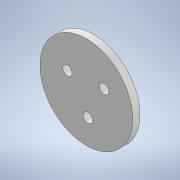
# Autodesk Inventor part: kółko
Saved by Autodesk Inventor 2022 (Build 260153000, 153)
## iProperties
Created: 2023-01-20
Part Number: kółko
Material: Generic
Document SubType Name: Modeling
Designer: Kamil
Density: 1 g/cm^3
Appearance: Default
Mass: 5.3524 g
Surface Area: 36.816 cm^2
Volume: 5.3524 cm^3
Author: Kamil
Autodesk Inventor part; units mm, degrees
ref_plane "YZ Plane" through (0, 0, 0) normal (1, 0, 0) x (0, 1, 0)
ref_plane "XZ Plane" through (0, 0, 0) normal (0, 1, 0) x (-1, 0, 0)
ref_plane "XY Plane" through (0, 0, 0) normal (0, 0, 1) x (1, 0, 0)
sketch "Sketch1" plane through (0, 0, 0) normal (0, 0, 1) x (1, 0, 0)
  circle A0 centre (-0.671, 10.228) radius 3.5 projected
  circle A1 centre (-8.5222, -5.6951) radius 3.5 projected
  circle A2 centre (9.1932, -4.5329) radius 3.5 projected
  circle A3 centre (0, 0) radius 15 projected
  circle A4 centre (8.5222, 5.6951) radius 2 projected
  circle A5 centre (0.671, -10.228) radius 2 projected
  circle A6 centre (-9.1932, 4.5329) radius 2 projected
  circle A7 centre (20.0905, -24.1532) radius 3.75 projected
  circle A8 centre (-30.4505, 7.7314) radius 3.75 projected
  circle A9 centre (-2.0567, 31.3493) radius 3.75 projected
  circle A10 centre (-16.7628, -26.571) radius 3.75 projected
  circle A11 centre (29.1794, 11.6435) radius 3.75 projected
  circle A12 centre (0, 0) radius 23.3333 projected
  arc A13 (-39.4862, -1.0454) -> (-35.737, -7.6127) centre (-31.489, -0.8337) ccw projected
  arc A14 (-34.2512, -12.7254) -> (-35.737, -7.6127) centre (-37.861, -11.0021) ccw projected
  arc A15 (-34.2512, -12.7254) -> (-33.8969, -20.2792) centre (-27.0317, -16.172) ccw projected
  arc A16 (-33.8969, -20.2792) -> (36.2558, -15.6768) centre (0, 0) ccw projected
  arc A17 (36.2558, -15.6768) -> (35.6202, -8.1415) centre (28.9129, -12.5018) ccw projected
  arc A18 (36.4252, -2.8784) -> (35.6202, -8.1415) centre (38.9739, -5.9614) ccw projected
  arc A19 (36.4252, -2.8784) -> (39.2843, 4.1223) centre (31.328, 3.2874) ccw projected
  arc A20 (39.2843, 4.1223) -> (-39.4862, -1.0454) centre (0, 0) ccw projected
  line L0 (0, 23.3333) -> (0, 22.3333)
  circle A21 centre (0, 0) radius 22.3333
  point P0 (0, 0)
  dimension "d0" = 1
  constraints: 2 end point, 2 vertical alignment, 1 coincident, 1 vertical, 3 other
  measures "d0" distance of L0.start L0.end
extrude "Extrusion1" add sketch "Sketch1" along normal blind 3.5 contours A0 | A1 | A2 | A3 | A21
sketch "Sketch2" plane through (0, 0, 0) normal (0, 0, -1) x (-1, 0, 0)
  circle A0 centre (0, 0) radius 22.3333 projected
  circle A1 centre (-8.5222, 5.6951) radius 2 projected
  circle A2 centre (-0.671, -10.228) radius 2 projected
  circle A3 centre (9.1932, 4.5329) radius 2 projected
  circle A4 centre (-8.5222, 5.6951) radius 2.25
  circle A5 centre (9.1932, 4.5329) radius 2.25
  circle A6 centre (-0.671, -10.228) radius 2 projected
  circle A7 centre (-0.671, -10.228) radius 2.25
  point P0 (0, 0)
  dimension "d3" = 4.5
  dimension "d4" = 4.5
  dimension "d5" = 4.5
  constraints: 3 centre point, 3 coincident
  measures "d3" diameter of A4
  measures "d4" diameter of A5
  measures "d5" diameter of A7
extrude "Extrusion2" cut sketch "Sketch2" against normal through all contours A1 | A2 | A3 | A4 | A5 | A7
body "Solid1"
